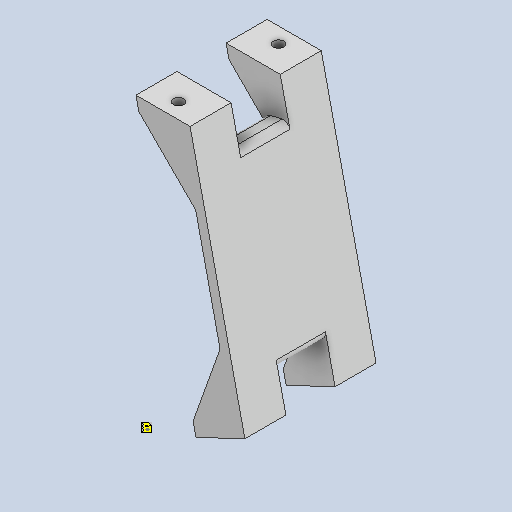
# Autodesk Inventor part: cam_krepl
Saved by Autodesk Inventor 2022 (Build 260153000, 153)
## iProperties
Created: 2022-12-28
Part Number: cam_krepl
Material: Типовые
Document SubType Name: Modeling
Designer: akapu
Density: 1 g/cm^3
Appearance: По умолчанию
Author: akapu
Autodesk Inventor part; units mm, degrees
ref_plane "YZ Plane" through (0, 0, 0) normal (1, 0, 0) x (0, 1, 0)
ref_plane "XZ Plane" through (0, 0, 0) normal (0, 1, 0) x (-1, 0, 0)
ref_plane "XY Plane" through (0, 0, 0) normal (0, 0, 1) x (1, 0, 0)
sketch "Эскиз1" plane through (0, 0, 0) normal (0, 0, 1) x (1, 0, 0)
  line L0 (-4.579, -9.6) -> (0.755, -9.6) projected
  line L1 (0.755, -8) -> (0.755, -9.6) projected
  line L2 (-4.579, -8) -> (0.755, -8) projected
  line L3 (-4.579, -8) -> (-4.579, -9.6) projected
  line L4 (-6, -9.6) -> (-9, -9.6) projected
  line L5 (-15.755, -9.6) -> (-10.421, -9.6) projected
  line L6 (-10.421, -8) -> (-10.421, -9.6) projected
  line L7 (-15.755, -8) -> (-10.421, -8) projected
  line L8 (-15.755, -8) -> (-15.755, -9.6) projected
  line L9 (22.0988, 32.6265) -> (54.8612, -112.7269) projected
  line L10 (22.0988, 32.6265) -> (19.1722, 31.9669) projected
  line L11 (51.9346, -113.3866) -> (19.1722, 31.9669) projected
  line L12 (54.8612, -112.7269) -> (51.9346, -113.3866) projected
  line L13 (0.755, -9.6) -> (9.1105, -46.67)
  line L14 (9.1105, -46.67) -> (17.466, -83.74)
  line L15 (0.755, -9.6) -> (-15.755, -9.6)
  line L16 (-15.755, -9.6) -> (-14.8755, -13.5021)
  line L17 (9.1105, -46.67) -> (6.1839, -47.3297)
  line L18 (6.1839, -47.3297) -> (-2.3203, -9.6)
  line L19 (-14.8755, -13.5021) -> (2.4686, -30.8462)
  line L20 (-14.8755, -13.5021) -> (9.6527, -13.5021) construction
  line L21 (11.3642, -86.6379) -> (8.6543, -87.9249)
  line L22 (17.466, -83.74) -> (2.5525, -90.8228)
  line L23 (2.5525, -90.8228) -> (1.6729, -86.9207)
  line L24 (1.6729, -86.9207) -> (9.8993, -63.8132)
  line L25 (6.1839, -47.3297) -> (14.6881, -85.0593)
  point P0 (0, 0)
  dimension "d0" = 38
  dimension "d1" = 4
  dimension "d2" = 3
  dimension "d3" = 45
  constraints: 26 end point, 5 symmetric about line, 4 point on line, 1 collinear, 1 equal length, 1 horizontal, 1 perpendicular
  measures "d0" distance of L13.end L14.end
  measures "d1" distance of L5.start L16.end
  measures "d2" distance of L13.end L17.end
  measures "d3" angle of L19 L20
extrude "Выдавливание1" add sketch "Эскиз1" along normal mid plane 40 contours L0 L18 L19 L16 L5 L15 L4 | L0 L13 L17 L18 | L14 L22 L25 L17 | L25 L22 L21 L23 L24
sketch "Эскиз2" plane through (0.755, -9.6, 20) normal (0.9755266, 0.2198816, 0) x (0, 0, -1)
  line L0 (27.5, 5.245) -> (12.5, 5.245) projected
  line L1 (12.5, 13.0492) -> (12.5, 5.245) projected
  line L2 (18.6, 13.0492) -> (12.5, 13.0492) projected
  line L3 (18.6, 13.0492) -> (18.6, 19.195) projected
  line L4 (21.4, 19.195) -> (18.6, 19.195) projected
  line L5 (21.4, 13.0492) -> (21.4, 19.195) projected
  line L6 (27.5, 13.0492) -> (21.4, 13.0492) projected
  line L7 (27.5, 13.0492) -> (27.5, 5.245) projected
  ellipse E0 centre (20, 17.0488) end of major axis (20.5, 17.0488) minor radius 0.4878 projected
  line L8 (27.5, 5.245) -> (27.5, -79.6302)
  line L9 (0, -79.6302) -> (40, -79.6302) projected
  line L10 (12.5, 5.245) -> (12.5, -79.6302)
  line L11 (12.5, -79.6302) -> (27.5, -79.6302)
  line L12 (94.75, -30.2019) -> (-70.28, -30.2019) projected
  line L13 (94.75, -45.7981) -> (-70.28, -45.7981) projected
  line L14 (40, 3.6302) -> (0, 3.6302) projected
  line L15 (27.5, 3.6302) -> (27.5, -6.3698)
  line L16 (27.5, -6.3698) -> (12.5, -6.3698)
  line L17 (27.5, -79.6302) -> (27.5, -69.6302)
  line L18 (27.5, -69.6302) -> (12.5, -69.6302)
  line L19 (27.5, -69.6302) -> (27.5, -64.6302)
  line L20 (27.5, -64.6302) -> (12.5, -64.6302)
  line L21 (27.5, -6.3698) -> (27.5, -11.3698)
  line L22 (27.5, -11.3698) -> (12.5, -11.3698)
  point P0 (20, 9.5311)
  point P1 (12.5, -30.2019)
  point P2 (27.5, -30.2019)
  point P3 (27.5, -45.7981)
  point P4 (12.5, -45.7981)
  point P5 (12.5, -79.6302)
  dimension "d26" = 10
  dimension "d27" = 10
  dimension "d28" = 5
  dimension "d29" = 5
  constraints: 22 end point, 11 point on line, 5 perpendicular, 2 vertical
  measures "d26" distance of L15.start L15.end
  measures "d27" distance of L8.end L17.end
  measures "d28" distance of L17.end L19.end
  measures "d29" distance of L15.end L21.end
extrude "Выдавливание2" cut sketch "Эскиз2" against normal blind 40 contours L8 L14 L10 L0 | L8 L16 L10 L14 | L8 L22 L10 L16 | L8 L18 L10 L20 | L8 L9 L10 L18
sketch "Эскиз3" plane through (-15.755, -9.6, 20) normal (0, 1, 0) x (1, 0, 0)
  circle A0 centre (8.255, 4.76) radius 1.5 projected
  circle A1 centre (8.255, 35.24) radius 1.5 projected
  circle A2 centre (8.255, 4.76) radius 1.5
  circle A3 centre (8.255, 35.24) radius 1.5
  point P0 (15.755, 20)
  constraints: 2 centre point, 2 coincident, 2 concentric
extrude "Выдавливание3" cut sketch "Эскиз3" against normal blind 40
sketch "Эскиз4" plane through (-15.755, -9.6, 20) normal (0, 1, 0) x (1, 0, 0)
  circle A0 centre (8.255, 4.76) radius 1.5 projected
  circle A1 centre (8.255, 4.76) radius 1.5
  circle A2 centre (8.255, 35.24) radius 1.5 projected
  circle A3 centre (8.255, 35.24) radius 1.5
  line L0 (8.255, 4.76) -> (8.255, 2.01)
  line L1 (8.255, 35.24) -> (8.255, 37.99)
  line L2 (6.6673, 2.01) -> (5.0796, 4.76)
  line L3 (5.0796, 4.76) -> (6.6673, 7.51)
  line L4 (6.6673, 7.51) -> (9.8427, 7.51)
  line L5 (9.8427, 7.51) -> (11.4304, 4.76)
  line L6 (11.4304, 4.76) -> (9.8427, 2.01)
  line L7 (9.8427, 2.01) -> (6.6673, 2.01)
  line L8 (9.8427, 37.99) -> (11.4304, 35.24)
  line L9 (11.4304, 35.24) -> (9.8427, 32.49)
  line L10 (9.8427, 32.49) -> (6.6673, 32.49)
  line L11 (6.6673, 32.49) -> (5.0796, 35.24)
  line L12 (5.0796, 35.24) -> (6.6673, 37.99)
  line L13 (6.6673, 37.99) -> (9.8427, 37.99)
  point P0 (15.755, 20)
  dimension "d10" = 2.75
  dimension "d11" = 2.75
  constraints: 28 end point, 4 coincident, 2 centre point, 2 midpoint, 2 vertical, 26 other
  measures "d10" distance of L0.start L0.end
  measures "d11" distance of L1.start L1.end
extrude "Выдавливание4" cut sketch "Эскиз4" against normal up to next contours A0 | A2 | L2 L3 L4 L5 L6 L7 | L8 L9 L10 L11 L12 L13
sketch "Эскиз5" plane through (-15.755, -9.6, 20) normal (0, 1, 0) x (1, 0, 0)
  line L0 (9.8427, 2.01) -> (11.4304, 4.76) projected
  line L1 (11.4304, 4.76) -> (9.8427, 2.01)
  line L2 (9.8427, 2.01) -> (6.6673, 2.01)
  line L3 (6.6673, 2.01) -> (5.0796, 4.76)
  line L4 (5.0796, 4.76) -> (6.6673, 7.51)
  line L5 (6.6673, 7.51) -> (9.8427, 7.51)
  line L6 (9.8427, 7.51) -> (11.4304, 4.76)
  line L7 (9.8427, 37.99) -> (11.4304, 35.24) projected
  line L8 (11.4304, 35.24) -> (9.8427, 32.49)
  line L9 (9.8427, 32.49) -> (6.6673, 32.49)
  line L10 (6.6673, 32.49) -> (5.0796, 35.24)
  line L11 (5.0796, 35.24) -> (6.6673, 37.99)
  line L12 (6.6673, 37.99) -> (9.8427, 37.99)
  line L13 (9.8427, 37.99) -> (11.4304, 35.24)
  circle A0 centre (8.255, 4.76) radius 1.5
  circle A1 centre (8.255, 35.24) radius 1.5
  circle A2 centre (8.255, 4.76) radius 1.6
  circle A3 centre (8.255, 35.24) radius 1.6
  point P0 (15.755, 20)
  dimension "d14" = 3
  dimension "d15" = 3
  dimension "d16" = 3.2
  dimension "d17" = 3.2
  constraints: 24 end point, 4 centre point, 4 coincident, 26 other
  measures "d14" diameter of A0
  measures "d15" diameter of A1
  measures "d16" diameter of A2
  measures "d17" diameter of A3
extrude "Выдавливание5" add sketch "Эскиз5" against normal blind 5 contours L2 L3 L4 L5 L6 L0 | L7 L8 L9 L10 L11 L12
sketch "Эскиз7" plane through (17.466, -83.74, 7.5) normal (0.4290008, -0.9033041, 0) x (0.9033041, 0.4290008, 0)
  ellipse E0 centre (9.2542, 7.74) end of major axis (9.2542, 6.24) minor radius 1.355 projected
  line L0 (0, 0) -> (0, 12.5) projected
  line L1 (0, -27.5) -> (-16.51, -27.5) projected
  line L2 (0, 12.5) -> (0, -27.5)
  ellipse E1 centre (-9.2542, 7.74) end of major axis (-9.2542, 6.24) minor radius 1.355
  line L3 (-9.2542, 7.74) -> (-9.2542, 10.49)
  line L4 (-7.6665, 10.49) -> (-6.0788, 7.74)
  line L5 (-6.0788, 7.74) -> (-7.6665, 4.99)
  line L6 (-7.6665, 4.99) -> (-10.8419, 4.99)
  line L7 (-10.8419, 4.99) -> (-12.4297, 7.74)
  line L8 (-12.4297, 7.74) -> (-10.8419, 10.49)
  line L9 (-10.8419, 10.49) -> (-7.6665, 10.49)
  line L10 (0, -7.5) -> (-16.51, -7.5)
  line L11 (-7.6665, -25.49) -> (-6.0788, -22.74)
  line L12 (-6.0788, -22.74) -> (-7.6665, -19.99)
  line L13 (-7.6665, -19.99) -> (-10.8419, -19.99)
  line L14 (-10.8419, -19.99) -> (-12.4297, -22.74)
  line L15 (-12.4297, -22.74) -> (-10.8419, -25.49)
  line L16 (-10.8419, -25.49) -> (-7.6665, -25.49)
  point P0 (20.1474, -7.5)
  point P1 (-9.2542, -25.49)
  dimension "d20" = 2.75
  constraints: 30 end point, 8 symmetric about line, 2 midpoint, 1 centre point, 1 coincident, 1 horizontal, 1 perpendicular, 1 vertical, 15 other
  measures "d20" distance of L3.start L3.end
extrude "Выдавливание6" cut sketch "Эскиз7" against normal up to next contours E1 | L4 L5 L6 L7 L8 L9 | L16 L15 L14 L13 L12 L11
sketch "Эскиз8" plane through (2.5525, -90.8228, -20) normal (0.4290008, -0.9033041, 0) x (0.9033041, 0.4290008, 0)
  line L0 (8.8435, 2.01) -> (10.4312, 4.76) projected
  line L1 (10.4312, 4.76) -> (8.8435, 2.01)
  line L2 (8.8435, 2.01) -> (5.6681, 2.01)
  line L3 (5.6681, 2.01) -> (4.0803, 4.76)
  line L4 (4.0803, 4.76) -> (5.6681, 7.51)
  line L5 (5.6681, 7.51) -> (8.8435, 7.51)
  line L6 (8.8435, 7.51) -> (10.4312, 4.76)
  line L7 (8.8435, 32.49) -> (10.4312, 35.24) projected
  line L8 (10.4312, 35.24) -> (8.8435, 32.49)
  line L9 (8.8435, 32.49) -> (5.6681, 32.49)
  line L10 (5.6681, 32.49) -> (4.0803, 35.24)
  line L11 (4.0803, 35.24) -> (5.6681, 37.99)
  line L12 (5.6681, 37.99) -> (8.8435, 37.99)
  line L13 (8.8435, 37.99) -> (10.4312, 35.24)
  circle A0 centre (7.2558, 4.76) radius 1.6
  circle A1 centre (7.2558, 35.24) radius 1.6
  point P0 (36.6574, 20)
  point P1 (8.8435, 32.49)
  point P2 (8.8435, 2.01)
  dimension "d23" = 3.2
  constraints: 24 end point, 2 centre point, 2 coincident, 26 other
  measures "d23" diameter of A0
extrude "Выдавливание7" add sketch "Эскиз8" against normal blind 5
fillet "Сопряжение1" radius 2 4 edges at (6.0374, -74.661, 0) (-5.6736, -22.704, 0) (3.255, -20.6915, 0) (14.966, -72.6485, 0)
